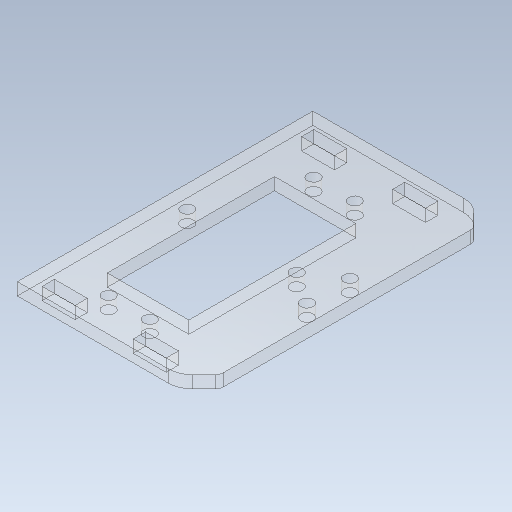
# Autodesk Inventor part: Dock bot1 V2
Saved by Autodesk Inventor 2020.3 (Build 243373000, 373)
## iProperties
Created: 2017-03-29
Part Number: Dock bot1 V2
Material: Acrylic
Document SubType Name: Modeling
Designer: Nanjar
Density: 1.188 g/cm^3
Appearance: Transparent - Clear
Mass: 7.78838 g
Surface Area: 58.9894 cm^2
Volume: 6.55588 cm^3
Author: Nanjar
Autodesk Inventor part; units mm, degrees
ref_plane "YZ Plane" through (0, 0, 0) normal (1, 0, 0) x (0, 1, 0)
ref_plane "XZ Plane" through (0, 0, 0) normal (0, 1, 0) x (-1, 0, 0)
ref_plane "XY Plane" through (0, 0, 0) normal (0, 0, 1) x (1, 0, 0)
sketch "Sketch1" plane through (0, 0, 0) normal (0, 1, 0) x (-1, 0, 0)
  circle A0 centre (-7.7007, -5.199) radius 1.5
  circle A1 centre (0, 0) radius 1.5
  circle A2 centre (-7.6993, 5.201) radius 1.5
  circle A3 centre (26.6, -0.0035) radius 1.5
  line L0 (31.9825, -36.8891) -> (31.9923, 36.8689)
  line L1 (-6.1404, -36.884) -> (31.9825, -36.8891)
  line L2 (-6.1306, 36.8689) -> (-12.1681, 30.833)
  line L3 (-12.1681, -30.8547) -> (-6.1404, -36.884)
  line L4 (22.9017, 23.1133) -> (22.9017, -17.4867)
  line L5 (3.1017, -17.4867) -> (3.1017, 23.1133)
  circle A4 centre (18.0017, -22.0763) radius 1.5
  circle A5 centre (18.0017, 27.7029) radius 1.5
  circle A6 centre (8.0017, -22.0763) radius 1.5
  circle A7 centre (8.0017, 27.7029) radius 1.5
  line L6 (-12.1681, 30.833) -> (-12.1681, -30.8547)
  line L7 (22.9017, 23.1133) -> (3.1017, 23.1133)
  line L8 (22.9017, -17.4867) -> (3.1017, -17.4867)
  line L9 (-6.1306, 36.8689) -> (31.9923, 36.8689)
  constraints: 21 end point, 8 centre point, 1 horizontal, 1 parallel, 1 perpendicular, 1 vertical
extrude "Extrusion1" add sketch "Sketch1" along normal blind 3
move faces "Move1" translate (0, 0, -0.995) faces at (-19.2846, 1, 36.8689)
move faces "Move2" translate (-0.0001, 0, 0.995) faces at (-6.5673, 2, -36.8857)
fillet "Fillet1" radius 6 2 edges at (7.1259, 1.5, 35.8739) (7.1352, 1.5, -35.8889)
fillet "Fillet2" radius 2 2 edges at (12.1681, 1.5, -30.8547) (12.1681, 1.5, 30.833)
sketch "Sketch4" plane through (0, 3, 0) normal (0, 1, 0) x (1, 0, 0)
  line L0 (2.1398, 32.1316) -> (2.1394, 29.1316)
  line L1 (2.1394, 29.1316) -> (-5.8606, 29.1327)
  line L2 (-5.8602, 32.1327) -> (2.1398, 32.1316)
  line L3 (-5.8602, 32.1327) -> (-5.8606, 29.1327)
  line L4 (-27.9915, -30.8644) -> (-27.9919, -33.8644)
  line L5 (-19.9915, -30.8654) -> (-19.9919, -33.8654)
  line L6 (-19.9919, -33.8654) -> (-27.9919, -33.8644)
  line L7 (-27.9915, -30.8644) -> (-19.9915, -30.8654)
  line L8 (-5.8686, -30.8673) -> (-5.869, -33.8673)
  line L9 (-5.8686, -30.8673) -> (2.1314, -30.8684)
  line L10 (2.1314, -30.8684) -> (2.131, -33.8684)
  line L11 (2.131, -33.8684) -> (-5.869, -33.8673)
  line L12 (-27.9832, 32.1356) -> (-19.9836, 32.1356)
  line L13 (-19.9836, 29.1346) -> (-27.9832, 29.1346)
  line L14 (-27.9832, 29.1346) -> (-27.9832, 32.1356)
  line L15 (-19.9836, 32.1356) -> (-19.9836, 29.1346)
  constraints: 32 end point, 1 horizontal, 1 parallel, 1 vertical
extrude "Extrusion2" cut sketch "Sketch4" against normal up to next
body "Solid1"
